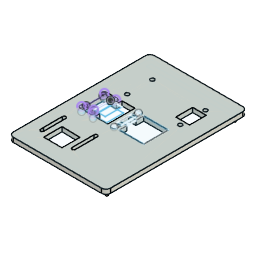
Lid and Case (Autodesk Fusion 360 archive; units mm, degrees)
design "Sensor Insert"
part number: 2026-04-01-18-16-49-366
Autodesk Fusion 360 part; units mm, degrees
sketch "Sketch5" plane through (0, 0, 0) normal (0, 0, 1) x (1, 0, 0)
  line L0 (3, 0) -> (61, 0)
  line L1 (64, 3) -> (64, 90)
  line L2 (61, 93) -> (3, 93)
  line L3 (0, 90) -> (0, 3)
  arc A0 (0, 3) -> (3, 0) centre (3, 3) ccw
  arc A1 (3, 93) -> (0, 90) centre (3, 90) ccw
  arc A2 (64, 90) -> (61, 93) centre (61, 90) ccw
  arc A3 (61, 0) -> (64, 3) centre (61, 3) ccw
  point P0 (64, 0)
  point P1 (0, 93)
  dimension "d27" = 64
  dimension "d28" = 93
  dimension "d29" = 3
  constraint horizontal L0
  constraint vertical L1
  constraint horizontal L2
  constraint vertical L3
  constraint coincident origin L0
  constraint coincident origin L3
  constraint tangent L0 A0
  constraint tangent L3 A0
  constraint coincident P1 L2
  constraint coincident P1 L3
  constraint tangent L2 A1
  constraint tangent L3 A1
  constraint equal A0 A1
  constraint tangent L1 A2
  constraint tangent L2 A2
  constraint equal A0 A2
  constraint coincident P0 L0
  constraint coincident P0 L1
  constraint tangent L0 A3
  constraint tangent L1 A3
  constraint equal A0 A3
  measures "d27" distance of origin P0
  measures "d28" distance of origin P1
  measures "d29" radius of A0
extrude "Extrude5" add sketch "Sketch5" along normal blind 3
sketch "Sketch6" plane through (0, 0, 0) normal (0, 0, -1) x (1, 0, 0)
  arc A0 (64, -3) -> (61, 0) centre (61, -3) ccw
  line L0 (61, 0) -> (3, 0)
  arc A1 (3, 0) -> (0, -3) centre (3, -3) ccw
  line L1 (0, -3) -> (0, -90)
  arc A2 (0, -90) -> (3, -93) centre (3, -90) ccw
  line L2 (3, -93) -> (61, -93)
  arc A3 (61, -93) -> (64, -90) centre (61, -90) ccw
  line L3 (64, -90) -> (64, -3)
  line L4 (3, -3) -> (61, -3)
  line L5 (61, -3) -> (61, -90)
  line L6 (61, -90) -> (3, -90)
  line L7 (3, -90) -> (3, -3)
  line L8 (3.5, -3) -> (60.5, -3)
  line L9 (60.5, -3) -> (60.5, -6)
  line L10 (60.5, -6) -> (3.5, -6)
  line L11 (3.5, -6) -> (3.5, -3)
  line L12 (3.5, -90) -> (60.5, -90)
  line L13 (60.5, -90) -> (60.5, -87)
  line L14 (60.5, -87) -> (3.5, -87)
  line L15 (3.5, -87) -> (3.5, -90)
  dimension "d32" = 58
  dimension "d33" = 87
  dimension "d34" = 3
  dimension "d35" = 3
  dimension "d36" = 57
  dimension "d37" = 3
  dimension "d38" = 0.5
  dimension "d39" = 57
  dimension "d40" = 3
  dimension "d151" = 0.5
  constraint horizontal L4
  constraint vertical L5
  constraint horizontal L6
  constraint vertical L7
  constraint horizontal L8
  constraint vertical L9
  constraint horizontal L10
  constraint vertical L11
  constraint coincident L4 L8.start
  constraint horizontal L12
  constraint vertical L13
  constraint horizontal L14
  constraint vertical L15
  constraint coincident L6 L12.start
  measures "d32" distance of A1.centre A0.centre
  measures "d33" distance of A1.centre A2.centre
  measures "d34" distance of L1 L7
  measures "d35" distance of L0 L4
  measures "d36" distance of L8.start L8.end
  measures "d37" distance of L8.start L10.end
  measures "d38" distance of L7 L11
  measures "d39" distance of L12.start L12.end
  measures "d40" distance of L12.start L14.end
  measures "d151" distance of L7 L15
extrude "Extrude6" add sketch "Sketch6" along normal blind 4 contours L4 L8 L9 L10 L11 | L6 L12 L13 L14 L15
sketch "Sketch8" plane through (0, 0, 0) normal (0, 0, -1) x (1, 0, 0)
  line L0 (3.5, -6) -> (3.5, -3)
  line L1 (3.5, -3) -> (60.5, -3)
  line L2 (60.5, -3) -> (60.5, -6)
  line L3 (60.5, -6) -> (3.5, -6)
  line L4 (3.5, -87) -> (60.5, -87)
  line L5 (60.5, -87) -> (60.5, -90)
  line L6 (60.5, -90) -> (3.5, -90)
  line L7 (3.5, -90) -> (3.5, -87)
  arc A0 (64, -3) -> (61, 0) centre (61, -3) ccw
  line L8 (61, 0) -> (3, 0)
  arc A1 (3, 0) -> (0, -3) centre (3, -3) ccw
  line L9 (0, -3) -> (0, -90)
  arc A2 (0, -90) -> (3, -93) centre (3, -90) ccw
  line L10 (3, -93) -> (61, -93)
  arc A3 (61, -93) -> (64, -90) centre (61, -90) ccw
  line L11 (64, -90) -> (64, -3)
  circle A4 centre (15.94, -61.99) radius 1.27
  circle A5 centre (15.94, -78.61) radius 1.27
  circle A6 centre (50.9, -78.61) radius 1.27
  circle A7 centre (50.9, -61.99) radius 1.27
  line L12 (64, -81) -> (0, -81)
  line L13 (0, -81) -> (0, -59.6)
  line L14 (0, -59.6) -> (64, -59.6)
  line L15 (64, -59.6) -> (64, -81)
  dimension "d52" = 2.54
  dimension "d55" = 2.54
  dimension "d58" = 2.54
  dimension "d61" = 2.54
  dimension "d85" = 64
  dimension "d86" = 21.4
  dimension "d87" = 6
  dimension "d92" = 2.39
  dimension "d93" = 2.39
  dimension "d96" = 2.39
  dimension "d97" = 15.94
  dimension "d98" = 2.39
  dimension "d99" = 15.94
  dimension "d100" = 50.9
  dimension "d101" = 50.9
  constraint horizontal L12
  constraint vertical L13
  constraint horizontal L14
  constraint vertical L15
  constraint coincident L11 L12.start
  measures "d52" diameter of A4
  measures "d55" diameter of A5
  measures "d58" diameter of A6
  measures "d61" diameter of A7
  measures "d85" distance of L12.start L12.end
  measures "d86" distance of L12.start L14.end
  measures "d87" distance of L4 L12
  measures "d92" distance of A7.centre L14
  measures "d93" distance of A6.centre L12
  measures "d96" distance of A5.centre L12
  measures "d97" distance of A5.centre L13
  measures "d98" distance of A4.centre L14
  measures "d99" distance of A4.centre L13
  measures "d100" distance of A6.centre L13
  measures "d101" distance of A7.centre L13
extrude "Extrude8" cut sketch "Sketch8" against normal blind 3 contours A4 | A5 | A6 | A7
sketch "Sketch9" plane through (0, 0, 0) normal (0, 0, -1) x (1, 0, 0)
  circle A0 centre (50.9, -61.99) radius 1.27
  circle A1 centre (50.9, -78.61) radius 1.27
  circle A2 centre (15.94, -61.99) radius 1.27
  circle A3 centre (15.94, -78.61) radius 1.27
  line L0 (3.5, -6) -> (3.5, -3)
  line L1 (3.5, -3) -> (60.5, -3)
  line L2 (60.5, -3) -> (60.5, -6)
  line L3 (60.5, -6) -> (3.5, -6)
  line L4 (3.5, -87) -> (60.5, -87)
  line L5 (60.5, -87) -> (60.5, -90)
  line L6 (60.5, -90) -> (3.5, -90)
  line L7 (3.5, -90) -> (3.5, -87)
  arc A4 (64, -3) -> (61, 0) centre (61, -3) ccw
  line L8 (61, 0) -> (3, 0)
  arc A5 (3, 0) -> (0, -3) centre (3, -3) ccw
  line L9 (0, -3) -> (0, -90)
  arc A6 (0, -90) -> (3, -93) centre (3, -90) ccw
  line L10 (3, -93) -> (61, -93)
  arc A7 (61, -93) -> (64, -90) centre (61, -90) ccw
  line L11 (64, -90) -> (64, -3)
  circle A8 centre (8, -40) radius 1.27
  circle A9 centre (8, -55) radius 1.27
  circle A10 centre (15.5, -40) radius 1.27
  circle A11 centre (15.5, -55) radius 1.27
  line L12 (9, -42) -> (14, -42)
  line L13 (14, -42) -> (14, -53)
  line L14 (14, -53) -> (9, -53)
  line L15 (9, -53) -> (9, -42)
  line L16 (14, -53) -> (22.5, -53)
  line L17 (22.5, -53) -> (22.5, -42)
  line L18 (22.5, -42) -> (14, -42)
  line L19 (14, -42) -> (14, -53)
  dimension "d70" = 2.54
  dimension "d73" = 2.54
  dimension "d76" = 2.54
  dimension "d79" = 2.54
  constraint horizontal L12
  constraint vertical L13
  constraint horizontal L14
  constraint vertical L15
  constraint horizontal L16
  constraint vertical L17
  constraint horizontal L18
  constraint vertical L19
  measures "d70" diameter of A8
  measures "d73" diameter of A9
  measures "d76" diameter of A10
  measures "d79" diameter of A11
extrude "Extrude9" cut sketch "Sketch9" against normal blind 3 contours A8 | A9 | A10 | A11 | L12 L13 L14 L15 L19
fillet "Fillet5" radius 1.5 4 edges at (32, 3, -4) (32, 6, -4) (32, 87, -4) (32, 90, -4)
sketch "Sketch11" plane through (0, 0, 3) normal (0, 0, 1) x (-1, 0, 0)
  circle A0 centre (-50.9, -61.99) radius 1.27
  circle A1 centre (-50.9, -78.61) radius 1.27
  circle A2 centre (-15.94, -61.99) radius 1.27
  circle A3 centre (-15.94, -78.61) radius 1.27
  arc A4 (-61, 0) -> (-64, -3) centre (-61, -3) ccw
  line L0 (-64, -3) -> (-64, -90)
  arc A5 (-64, -90) -> (-61, -93) centre (-61, -90) ccw
  line L1 (-61, -93) -> (-3, -93)
  arc A6 (-3, -93) -> (0, -90) centre (-3, -90) ccw
  line L2 (0, -90) -> (0, -3)
  arc A7 (0, -3) -> (-3, 0) centre (-3, -3) ccw
  line L3 (-3, 0) -> (-61, 0)
  line L4 (-14, -53) -> (-14, -42)
  line L5 (-14, -42) -> (-9, -42)
  line L6 (-9, -42) -> (-9, -53)
  line L7 (-9, -53) -> (-14, -53)
  circle A8 centre (-15.5, -40) radius 1.27
  circle A9 centre (-8, -55) radius 1.27
  circle A10 centre (-8, -40) radius 1.27
  circle A11 centre (-15.5, -55) radius 1.27
sketch "Sketch12" plane through (0, 0, 3) normal (0, 0, 1) x (-1, 0, 0)
  circle A0 centre (-8.497, -15.503) radius 1.1
  circle A1 centre (-8.497, -28.003) radius 1.1
  circle A2 centre (-29.297, -28.003) radius 1.1
  line L0 (-12.997, -10.1) -> (-12.997, -22.1)
  line L1 (-12.997, -22.1) -> (-24.997, -21.8275)
  line L2 (-24.997, -21.8275) -> (-24.997, -10.1)
  line L3 (-24.997, -10.1) -> (-12.997, -10.1)
  line L4 (-8, -41.3) -> (-15.5, -41.3)
  line L5 (-15.5, -41.3) -> (-15.5, -38.7)
  line L6 (-15.5, -38.7) -> (-8, -38.7)
  line L7 (-8, -38.7) -> (-8, -41.3)
  line L8 (-15.5, -56.3) -> (-8, -56.3)
  line L9 (-8, -56.3) -> (-8, -53.7)
  line L10 (-8, -53.7) -> (-15.5, -53.7)
  line L11 (-15.5, -53.7) -> (-15.5, -56.3)
  line L12 (-54, -76) -> (-45, -76)
  line L13 (-45, -76) -> (-45, -65)
  line L14 (-45, -65) -> (-54, -65)
  line L15 (-54, -65) -> (-54, -76)
  line L16 (-7.3994, -28.077) -> (-9.5994, -28.077)
  line L17 (-9.5994, -28.077) -> (-9.5994, -13.503)
  line L18 (-9.5994, -13.503) -> (-7.3994, -13.503)
  line L19 (-7.3994, -13.503) -> (-7.3994, -28.077)
  line L20 (-28.1994, -28.077) -> (-30.3994, -28.077)
  line L21 (-30.3994, -28.077) -> (-30.3994, -13.503)
  line L22 (-30.3994, -13.503) -> (-28.1994, -13.503)
  line L23 (-28.1994, -13.503) -> (-28.1994, -28.077)
  arc A3 (-7.3994, -13.503) -> (-9.5994, -13.503) centre (-8.4994, -13.503) ccw
  arc A4 (-28.1994, -13.503) -> (-30.3994, -13.503) centre (-29.2994, -13.503) ccw
  line L24 (-3, 0) -> (-61, 0)
  dimension "d108" = 2.2
  dimension "d114" = 2.2
  dimension "d117" = 2.2
  dimension "d120" = 12
  dimension "d121" = 12
  dimension "d143" = 2.2
  dimension "d144" = 14.574
  dimension "d145" = 2.2
  dimension "d146" = 14.574
  dimension "d153" = 10.1
  constraint horizontal L4
  constraint vertical L5
  constraint horizontal L6
  constraint vertical L7
  constraint horizontal L8
  constraint vertical L9
  constraint horizontal L10
  constraint vertical L11
  constraint horizontal L12
  constraint vertical L13
  constraint horizontal L14
  constraint vertical L15
  constraint horizontal L16
  constraint vertical L17
  constraint horizontal L18
  constraint vertical L19
  constraint coincident A1 L16.start
  constraint horizontal L20
  constraint vertical L21
  constraint horizontal L22
  constraint vertical L23
  constraint coincident A2 L20.start
  constraint tangent L17 A3
  measures "d108" diameter of A0
  measures "d114" diameter of A1
  measures "d117" diameter of A2
  measures "d120" distance of L0.start L0.end
  measures "d121" distance of L0.start L2.end
  measures "d143" distance of L16.start L16.end
  measures "d144" distance of L16.start L18.end
  measures "d145" distance of L20.start L20.end
  measures "d146" distance of L20.start L22.end
  measures "d153" distance of L3 L24
extrude "Extrude10" cut sketch "Sketch12" against normal blind 3 contours A0 L19 | A0 L19 | A0 A1 L16 L17 L18 L19 | L18 A3 | A1 L16 L19 | A1 L19 | A1 L16 | A2 L23 | A2 L20 | A2 L20 L23 | A2 L20 L21 L22 L23 | L22 A4 | L0 L1 L2 L3
sketch "Sketch13" plane through (0, 0, 3) normal (0, 0, 1) x (-1, 0, 0)
  line L0 (-29, -55.0268) -> (-31.8, -55.0268)
  line L1 (-31.8, -55.0268) -> (-31.8, -39.0268)
  line L2 (-31.8, -39.0268) -> (-29, -39.0268)
  line L3 (-29, -39.0268) -> (-29, -55.0268)
  arc A0 (-31.8, -55.0268) -> (-29, -55.0268) centre (-30.4, -55.0268) ccw
  arc A1 (-29, -39.0268) -> (-31.8, -39.0268) centre (-30.4, -39.0268) ccw
  line L4 (-33.8, -55) -> (-49.8, -55)
  line L5 (-49.8, -55) -> (-49.8, -39)
  line L6 (-49.8, -39) -> (-33.8, -39)
  line L7 (-33.8, -39) -> (-33.8, -55)
  line L8 (-14, -42) -> (-14, -53)
  line L9 (-29, -50.0268) -> (-31.8, -50.0268)
  line L10 (-31.8, -50.0268) -> (-31.8, -44.0268)
  line L11 (-31.8, -44.0268) -> (-29, -44.0268)
  line L12 (-29, -44.0268) -> (-29, -50.0268)
  line L13 (-29, -52.0268) -> (-31.8, -52.0268)
  line L14 (-31.8, -52.0268) -> (-31.8, -42.0268)
  line L15 (-31.8, -42.0268) -> (-29, -42.0268)
  line L16 (-29, -42.0268) -> (-29, -52.0268)
  line L17 (-31.8, -50.0268) -> (-33.8, -50.0268)
  line L18 (-33.8, -50.0268) -> (-33.8, -44.0268)
  line L19 (-33.8, -44.0268) -> (-31.8, -44.0268)
  line L20 (-31.8, -44.0268) -> (-31.8, -50.0268)
  line L21 (-14, -53) -> (-21.5354, -53)
  line L22 (-21.5354, -53) -> (-21.5354, -42)
  line L23 (-21.5354, -42) -> (-14, -42)
  line L24 (-14, -42) -> (-14, -53)
  dimension "d126" = 2.8
  dimension "d127" = 16
  dimension "d128" = 16
  dimension "d129" = 16
  dimension "d130" = 2
  dimension "d133" = 15
  dimension "d134" = 6
  dimension "d135" = 5
  dimension "d136" = 2.8
  dimension "d137" = 10
  dimension "d138" = 3
  constraint horizontal L0
  constraint vertical L1
  constraint horizontal L2
  constraint vertical L3
  constraint tangent L1 A0
  constraint tangent L1 A1
  constraint horizontal L4
  constraint vertical L5
  constraint horizontal L6
  constraint vertical L7
  constraint horizontal L9
  constraint vertical L10
  constraint horizontal L11
  constraint vertical L12
  constraint coincident L3 L9.start
  constraint horizontal L13
  constraint vertical L14
  constraint horizontal L15
  constraint vertical L16
  constraint coincident L3 L13.start
  constraint horizontal L17
  constraint vertical L18
  constraint horizontal L19
  constraint vertical L20
  constraint coincident L7 L18.end
  constraint horizontal L21
  constraint vertical L22
  constraint horizontal L23
  constraint vertical L24
  constraint coincident L8.end L21.start
  measures "d126" distance of L0.start L0.end
  measures "d127" distance of L0.start L2.end
  measures "d128" distance of L4.start L4.end
  measures "d129" distance of L4.start L6.end
  measures "d130" distance of L1 L7
  measures "d133" distance of L3 L8
  measures "d134" distance of L9.start L11.end
  measures "d135" distance of L0 L9
  measures "d136" distance of L10.end L11.end
  measures "d137" distance of L13.start L15.end
  measures "d138" distance of L2 L15
extrude "Extrude12" cut sketch "Sketch13" against normal blind 3 contours L0 A0 | L0 L1 L3 L13 | L1 L3 L9 L10 L11 L12 L14 L16 L20 | L1 L7 L10 L14 L17 L18 L19 L20 | L4 L5 L6 L7 L18 | L1 L2 L3 L15 | L2 A1
extrude "Extrude13" cut sketch "Sketch12" against normal blind 3 contours L4 L5 L6 L7 | L8 L9 L10 L11 | L12 L13 L14 L15
extrude "Extrude14" cut sketch "Sketch13" against normal blind 3 contours L8 L21 L22 L23 L24
sketch "Sketch14" plane through (0, 0, 3) normal (0, 0, 1) x (-1, 0, 0)
  line L0 (-18, -38.7) -> (-26.5, -38.7)
  line L1 (-26.5, -38.7) -> (-26.5, -56.5)
  line L2 (-26.5, -56.5) -> (-18, -56.5)
  line L3 (-18, -56.5) -> (-18, -38.7)
  constraint horizontal L0
  constraint vertical L1
  constraint horizontal L2
  constraint vertical L3
extrude "Extrude15" cut sketch "Sketch14" against normal blind 3
sketch "Sketch15" plane through (0, 0, 3) normal (0, 0, 1) x (-1, 0, 0)

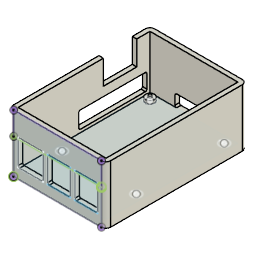
design "Case"
part number: 2026-04-01-16-26-12-971
Autodesk Fusion 360 part; units mm, degrees
sketch "Sketch1" plane through (0, 0, 0) normal (0, 0, 1) x (1, 0, 0)
  line L0 (3, 0) -> (61, 0)
  line L1 (64, 3) -> (64, 90)
  line L2 (61, 93) -> (3, 93)
  line L3 (0, 90) -> (0, 3)
  arc A0 (3, 93) -> (0, 90) centre (3, 90) ccw
  arc A1 (64, 90) -> (61, 93) centre (61, 90) ccw
  arc A2 (61, 0) -> (64, 3) centre (61, 3) ccw
  arc A3 (0, 3) -> (3, 0) centre (3, 3) ccw
  point P0 (64, 0)
  point P1 (0, 93)
  dimension "d1" = 64
  dimension "d2" = 93
  dimension "d3" = 3
  dimension "d4" = 3
  constraint horizontal L0
  constraint vertical L1
  constraint horizontal L2
  constraint vertical L3
  constraint coincident P1 L2
  constraint coincident P1 L3
  constraint tangent L2 A0
  constraint tangent L3 A0
  constraint tangent L1 A1
  constraint tangent L2 A1
  constraint equal A0 A1
  constraint coincident P0 L0
  constraint coincident P0 L1
  constraint tangent L0 A2
  constraint tangent L1 A2
  constraint equal A0 A2
  constraint coincident origin L0
  constraint coincident origin L3
  constraint tangent L0 A3
  constraint tangent L3 A3
  measures "d1" distance of origin P0
  measures "d2" distance of origin P1
  measures "d3" radius of A0
  measures "d4" radius of A3
extrude "Extrude1" add sketch "Sketch1" along normal blind 3
sketch "Sketch4" plane through (0, 0, 3) normal (0, 0, 1) x (-1, 0, 0)
  arc A0 (0, -3) -> (-3, 0) centre (-3, -3) ccw
  line L0 (-3, 0) -> (-61, 0)
  arc A1 (-61, 0) -> (-64, -3) centre (-61, -3) ccw
  line L1 (-64, -3) -> (-64, -90)
  arc A2 (-64, -90) -> (-61, -93) centre (-61, -90) ccw
  line L2 (-61, -93) -> (-3, -93)
  arc A3 (-3, -93) -> (0, -90) centre (-3, -90) ccw
  line L3 (0, -90) -> (0, -3)
  line L4 (-3, -3) -> (-61, -3)
  line L5 (-61, -3) -> (-61, -90)
  line L6 (-61, -90) -> (-3, -90)
  line L7 (-3, -90) -> (-3, -3)
  dimension "d11" = 58
  dimension "d12" = 87
  dimension "d13" = 3
  dimension "d14" = 3
  constraint horizontal L4
  constraint vertical L5
  constraint horizontal L6
  constraint vertical L7
  measures "d11" distance of A0.centre A1.centre
  measures "d12" distance of A0.centre A3.centre
  measures "d13" distance of L3 L7
  measures "d14" distance of L0 L4
extrude "Extrude2" add sketch "Sketch4" along normal blind 35
sketch "Sketch5" plane through (0, 0, 0) normal (0, -1, 0) x (1, 0, 0)
  line L0 (3, 0) -> (61, 0)
  line L1 (61, 0) -> (61, 23)
  line L2 (3, 23) -> (61, 23)
  line L3 (6, 6.8) -> (22.5, 6.8)
  line L4 (22.5, 6.8) -> (22.5, 23.8)
  line L5 (22.5, 23.8) -> (6, 23.8)
  line L6 (6, 23.8) -> (6, 6.8)
  line L7 (3, 0) -> (3, 23)
  line L8 (25.5, 23.8) -> (40.45, 23.8)
  line L9 (40.45, 23.8) -> (40.45, 6.8)
  line L10 (40.45, 6.8) -> (25.5, 6.8)
  line L11 (25.5, 6.8) -> (25.5, 23.8)
  line L12 (43.45, 6.8) -> (58.4, 6.8)
  line L13 (58.4, 6.8) -> (58.4, 23.8)
  line L14 (58.4, 23.8) -> (43.45, 23.8)
  line L15 (43.45, 23.8) -> (43.45, 6.8)
  line L16 (3, 0) -> (61, 0)
  line L17 (61, 0) -> (61, 38)
  line L18 (61, 38) -> (3, 38)
  line L19 (3, 38) -> (3, 0)
  dimension "d21" = 16.5
  dimension "d22" = 17
  dimension "d23" = 3
  dimension "d26" = 14.95
  dimension "d27" = 17
  dimension "d29" = 14.95
  dimension "d30" = 17
  dimension "d31" = 3
  dimension "d34" = 3
  dimension "d45" = 6.8
  constraint horizontal L3
  constraint vertical L4
  constraint horizontal L5
  constraint vertical L6
  constraint horizontal L8
  constraint vertical L9
  constraint horizontal L10
  constraint vertical L11
  constraint horizontal L12
  constraint vertical L13
  constraint horizontal L14
  constraint vertical L15
  measures "d21" distance of L3.start L3.end
  measures "d22" distance of L3.start L5.end
  measures "d23" distance of L6 L7
  measures "d26" distance of L8.start L8.end
  measures "d27" distance of L8.start L10.end
  measures "d29" distance of L12.start L12.end
  measures "d30" distance of L12.start L14.end
  measures "d31" distance of L9 L15
  measures "d34" distance of L4 L11
  measures "d45" distance of L0 L3
extrude "Extrude4" cut sketch "Sketch5" against normal blind 3 contours L2 L4 L5 L6 | L2 L3 L4 L6 | L2 L12 L13 L15 | L2 L13 L14 L15 | L2 L8 L9 L11 | L2 L9 L10 L11
sketch "Sketch6" plane through (0, 0, 3) normal (0, 0, 1) x (-1, 0, 0)
  line L0 (-3, -3) -> (-61, -3)
  line L1 (-61, -3) -> (-61, -90)
  line L2 (-61, -90) -> (-3, -90)
  line L3 (-3, -90) -> (-3, -3)
  circle A0 centre (-7.5, -85.5) radius 1
  circle A1 centre (-7.5, -85.5) radius 3
  circle A2 centre (-56.5, -85.5) radius 1
  circle A3 centre (-56.5, -85.5) radius 3
  circle A4 centre (-56.5, -27.5) radius 1
  circle A5 centre (-56.5, -27.5) radius 3
  circle A6 centre (-7.5, -27.5) radius 1
  circle A7 centre (-7.5, -27.5) radius 3
  dimension "d35" = 2
  dimension "d36" = 4.5
  dimension "d37" = 4.5
  dimension "d38" = 6
  dimension "d59" = 2
  dimension "d60" = 4.5
  dimension "d61" = 4.5
  dimension "d62" = 6
  dimension "d63" = 2
  dimension "d64" = 4.5
  dimension "d65" = 58
  dimension "d66" = 6
  dimension "d67" = 2
  dimension "d68" = 4.5
  dimension "d69" = 58
  dimension "d70" = 6
  constraint concentric A0 A1
  constraint concentric A2 A3
  constraint concentric A4 A5
  constraint concentric A6 A7
  measures "d35" diameter of A0
  measures "d36" distance of L2 A0.centre
  measures "d37" distance of L3 A0.centre
  measures "d38" diameter of A1
  measures "d59" diameter of A2
  measures "d60" distance of L2 A2.centre
  measures "d61" distance of L1 A2.centre
  measures "d62" diameter of A3
  measures "d63" diameter of A4
  measures "d64" distance of L1 A4.centre
  measures "d65" distance of A2.centre A4.centre
  measures "d66" diameter of A5
  measures "d67" diameter of A6
  measures "d68" distance of L3 A6.centre
  measures "d69" distance of A0.centre A6.centre
  measures "d70" diameter of A7
extrude "Extrude6" cut sketch "Sketch6" against normal blind 3 contours A0 | A2 | A4 | A6
extrude "Extrude7" add sketch "Sketch6" along normal blind 0.5 contours A1
sketch "Sketch7" plane through (0, 0, 0) normal (-1, 0, 0) x (0, -1, 0)
  line L0 (-90, 0) -> (-3, 0)
  line L1 (-3, 0) -> (-3, 38)
  line L2 (-3, 38) -> (-90, 38)
  line L3 (-90, 38) -> (-90, 0)
  line L4 (-88, 5) -> (-43, 5)
  line L5 (-43, 5) -> (-43, 16)
  line L6 (-43, 16) -> (-88, 16)
  line L7 (-88, 16) -> (-88, 5)
  dimension "d46" = 45
  dimension "d47" = 11
  dimension "d50" = 5
  constraint horizontal L4
  constraint vertical L5
  constraint horizontal L6
  constraint vertical L7
  measures "d46" distance of L4.start L4.end
  measures "d47" distance of L4.start L6.end
  measures "d50" distance of L0 L4
extrude "Extrude8" cut sketch "Sketch7" against normal blind 3 contours L4 L5 L6 L7
sketch "Sketch8" plane through (0, 93, 0) normal (0, 1, 0) x (-1, 0, 0)
  line L0 (-61, 0) -> (-3, 0)
  line L1 (-3, 0) -> (-3, 38)
  line L2 (-3, 38) -> (-61, 38)
  line L3 (-61, 38) -> (-61, 0)
  line L4 (-44.5, 3) -> (-19.5, 3)
  line L5 (-19.5, 3) -> (-19.5, 11)
  line L6 (-19.5, 11) -> (-44.5, 11)
  line L7 (-44.5, 11) -> (-44.5, 3)
  line L8 (-3, 0) -> (-3, 23)
  line L9 (-3, 0) -> (-61, 0)
  dimension "d51" = 25
  dimension "d52" = 8
  dimension "d53" = 16.5
  dimension "d54" = 3
  constraint horizontal L4
  constraint vertical L5
  constraint horizontal L6
  constraint vertical L7
  measures "d51" distance of L4.start L4.end
  measures "d52" distance of L4.start L6.end
  measures "d53" distance of L5 L8
  measures "d54" distance of L4 L9
extrude "Extrude9" cut sketch "Sketch8" against normal blind 3 contours L4 L5 L6 L7
extrude "Extrude10" add 1 faces at (9.6751, 86.3269, 3.5) along direction (0, 0, 1) blind 1.5
extrude "Extrude11" add sketch "Sketch6" along normal blind 2 contours A3 | A5 | A7
extrude "Extrude13" add sketch "Sketch6" along normal blind 3 contours A4
extrude "Extrude14" add sketch "Sketch6" along normal blind 3 contours A0 | A2 | A6
sketch "Sketch11" plane through (0, 0, 0) normal (-1, 0, 0) x (0, -1, 0)
  line L0 (-43, 5) -> (-88, 5)
  line L1 (-88, 5) -> (-88, 16)
  line L2 (-88, 16) -> (-43, 16)
  line L3 (-43, 16) -> (-43, 5)
  line L4 (-90, 0) -> (-3, 0)
  line L5 (-3, 0) -> (-3, 38)
  line L6 (-3, 38) -> (-90, 38)
  line L7 (-90, 38) -> (-90, 0)
  line L8 (-81.3, 38) -> (-59.3, 38)
  line L9 (-59.3, 38) -> (-59.3, 22)
  line L10 (-59.3, 22) -> (-81.3, 22)
  line L11 (-81.3, 22) -> (-81.3, 38)
  dimension "d85" = 22
  dimension "d86" = 16
  dimension "d87" = 8.7
  constraint horizontal L8
  constraint vertical L9
  constraint horizontal L10
  constraint vertical L11
  constraint coincident L6 L8.start
  measures "d85" distance of L8.start L8.end
  measures "d86" distance of L8.start L10.end
  measures "d87" distance of L7 L11
extrude "Extrude15" cut sketch "Sketch11" against normal blind 3 contours L6 L8 L9 L10 L11
fillet "Fillet1" radius 1 1 edges at (1.5, 81.3, 22)
fillet "Fillet2" radius 1 21 edges at (1.5, 59.3, 22) (44.5, 91.5, 3) (44.5, 91.5, 11) (19.5, 91.5, 3) (19.5, 91.5, 11) (1.5, 43, 5) (6, 1.5, 6.8) (25.5, 1.5, 6.8) (43.45, 1.5, 6.8) (6, 1.5, 23.8) (25.5, 1.5, 23.8) (43.45, 1.5, 23.8) (40.45, 1.5, 23.8) (22.5, 1.5, 23.8) (58.4, 1.5, 23.8) (1.5, 88, 16) (1.5, 88, 5) (22.5, 1.5, 6.8) (40.45, 1.5, 6.8) (58.4, 1.5, 6.8) (1.5, 43, 16)
delete_face "DeleteFace1" 1 faces at (1, 80.5358, 22.0282)
delete_face "DeleteFace2" 1 faces at (1, 59.8, 22.134)
